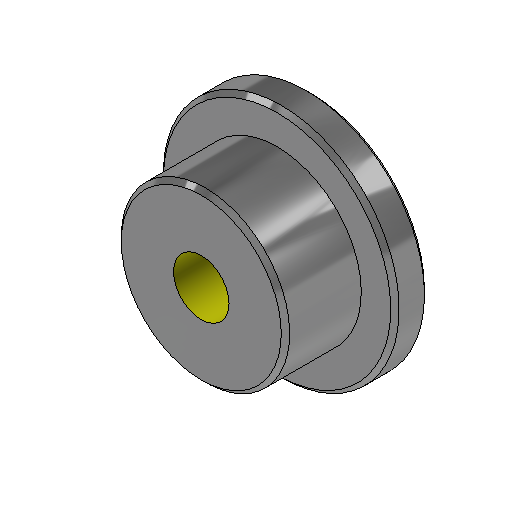
# Autodesk Inventor part: TL20240701-10110CV-006
Saved by Autodesk Inventor 2022.5 (Build 265521000, 521)
## iProperties
Category: DRIVE UNIT ASSY
Company: 현대 트랜시스(대유)
Created: 2023-02-21
Part Number: TL20240701-10110CV-006
Checked By: 김형민
Engr Approved By: 김시현
Material: S45C
Description: 0
Document SubType Name: Modeling
Mfg Approved By: 호상태
Designer: 박성규
Density: 7.87 g/cm^3
Appearance: Plating Chrome
Project: SW PJT
Stock Number: 006
User Status: 2 x18
DETAIL: Coveryor Assembly
M/C TITLE: MEa/NEa차종 시트조립라인
PARTS NAME: Bracket
SPECIFICATION: TA20221101-CV200000-015
DocNumber: 221118_Standard_v1
Folder: .\
VDS_Category: 엔지니어링
Detail Description: Processed products
Title: END CAP
Subject: SW차종 시트조립라인
Author: 박성규
Revision Number: A
Autodesk Inventor part; units mm, degrees
ref_plane "YZ Plane" through (0, 0, 0) normal (1, 0, 0) x (0, 1, 0)
ref_plane "XZ Plane" through (0, 0, 0) normal (0, 1, 0) x (-1, 0, 0)
ref_plane "XY Plane" through (0, 0, 0) normal (0, 0, 1) x (1, 0, 0)
sketch "Sketch11" plane through (0, 0, 0) normal (1, 0, 0) x (0, 1, 0)
  line L0 (0, -6.5) -> (0, 6.5)
  line L1 (0, -6.5) -> (14, -6.5)
  line L2 (14, -6.5) -> (14, -2.5)
  line L3 (14, -2.5) -> (10, -2.5)
  line L4 (10, -2.5) -> (10, 6.5)
  line L5 (10, 6.5) -> (0, 6.5)
  point P0 (0, 0)
  point P1 (0, 0)
  dimension "d50" = 20
  dimension "d51" = 28
  dimension "d52" = 4
  dimension "d53" = 13
  constraints: 12 end point, 3 perpendicular, 2 vertical, 1 coincident, 1 horizontal, 1 midpoint
  measures "d50" diameter of L4 L0
  measures "d51" diameter of L2 L0
  measures "d52" distance between parallel lines of L3 L1
  measures "d53" distance of L0.start L0.end
revolve "Revolution1" add sketch "Sketch11" angle 360 about axis through (0, 0, -6.5) along (0, 0, 1)
sketch "Sketch12" plane through (0, 0, -6.5) normal (0, 0, -1) x (-1, 0, 0)
  circle A0 centre (0, 0) radius 14 projected
  point P0 (0, 0)
  constraints: 1 coincident
hole "Hole4" at (0, 0, -6.5) direction (0, 0, 1) diameter 6.6 end through all counterbore diameter 11 counterbore depth 6.5 clearance for "Socket Head Cap Screw" size "M6" standard "TS Profile"
chamfer "Chamfer1" distance 0.5 angle 45 3 edges at (0, -10, 6.5) (0, -14, -2.5) (0, -14, -6.5)
body "Solid4"
